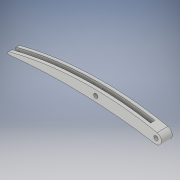
# Autodesk Inventor part: panto_legA
Saved by Autodesk Inventor 2017 (Build 210142000, 142)
## iProperties
Created: 2016-08-26
Part Number: panto_legA
Material: Generic
Document SubType Name: Modeling
Designer: Nic
Density: 1 g/cm^3
Appearance: Default
Author: Nic
Autodesk Inventor part; units mm, degrees
ref_plane "Work Plane1" through (0, 0, 0.75) normal (0, 0, 1) x (1, 0, 0)
ref_plane "YZ Plane" through (0, 0, 0) normal (1, 0, 0) x (0, 1, 0)
ref_plane "XZ Plane" through (0, 0, 0) normal (0, 1, 0) x (-1, 0, 0)
sketch "Sketch1" plane through (0, 0, 0) normal (0, 0, 1) x (1, 0, 0)
  circle A0 centre (68, 0) radius 1
  circle A1 centre (40.1612, 3) radius 1
  circle A2 centre (40.1612, 3) radius 2.5 construction
  arc A3 (-0.1519, 0.5805) -> (0.0642, -0.5966) centre (0, 0) ccw
  arc A4 (68.5003, 2.4494) -> (-0.1519, 0.5805) centre (38.1892, -145.9659) ccw
  arc A5 (67.5954, -2.467) -> (0.0642, -0.5966) centre (26.9372, -250.3803) ccw
  arc A6 (67.5954, -2.467) -> (68.5003, 2.4494) centre (68, 0) ccw
  arc A7 (38.0337, 4.313) -> (8.652, 1.3817) centre (38.1892, -145.9659) ccw
  arc A8 (37.9659, 1.8038) -> (8.652, 1.3817) centre (26.9372, -250.3803) ccw
  arc A9 (38.0337, 4.313) -> (37.9659, 1.8038) centre (40.1612, 3) ccw
  point P0 (40.1612, 6.5)
  dimension "d1" = 2
  dimension "d2" = 2
  dimension "d4" = 3
  dimension "d8" = 5
  dimension "d9" = 3.5
  dimension "d21" = 0.6
  dimension "d22" = 2.5
  dimension "d23" = 0
  dimension "d24" = 1.2
  dimension "d25" = 1.2
  dimension "d31" = 68
  dimension "d40" = 28
  constraints: 16 point on circle, 10 centre point, 6 tangent, 4 coincident, 2 concentric, 1 vertical alignment
  measures "d1" diameter of A0
  measures "d2" diameter of A1
  measures "d4" vertical distance of A0.centre A1.centre
  measures "d8" diameter of A2
  measures "d9" distance of A1.centre point (40.161, 6.5)
  measures "d21" radius of A3
  measures "d22" radius of A6
  measures "d23" vertical distance of point (0, 0) A0.centre
  measures "d24" radial gap between concentric circles of A5 A8
  measures "d25" radial gap between concentric circles of A4 A7
  measures "d31" distance of A0.centre point (0, 0)
  measures "d40" distance of A6.centre A1.centre
extrude "Extrusion1" add sketch "Sketch1" along normal blind 5 contours A4 A6 A5 A3 | A9 A8 A7
sketch "Sketch3" plane through (0, 0, 0) normal (0, 1, 0) x (-1, 0, 0)
  line L0 (4, 1.5) -> (-64, 1.5)
  line L1 (-64, 1.5) -> (-64, 3.5)
  line L2 (-64, 3.5) -> (4, 3.5)
  line L3 (4, 3.5) -> (4, 1.5)
  line L4 (-0.0642, 0) -> (-0.0642, 5) projected
  point P0 (0, 0)
  dimension "d34" = 1.5
  dimension "d35" = 4
  dimension "d36" = 2
  dimension "d37" = 68
  constraints: 8 end point, 2 parallel, 1 horizontal, 1 perpendicular
  measures "d34" distance from line of L0 point (0, 0)
  measures "d35" distance from line of L3 point (0, 0)
  measures "d36" distance between parallel lines of L2 L0
  measures "d37" distance from line of L2.end L1
extrude "Extrusion3" cut sketch "Sketch3" along normal through all both and the other way through all
body "Solid1"
